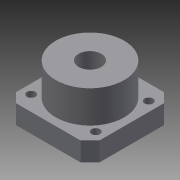
# Autodesk Inventor part: fk12
Saved by Autodesk Inventor 2014 (Build 180170000, 170)
## iProperties
Created: 2014-10-05
Part Number: fk12
Material: Generic
Document SubType Name: Modeling
Designer: Matthew
Density: 1 g/cm^3
Appearance: Default
Author: Matthew
Autodesk Inventor part; units mm, degrees
ref_plane "YZ Plane" through (0, 0, 0) normal (1, 0, 0) x (0, 1, 0)
ref_plane "XZ Plane" through (0, 0, 0) normal (0, 1, 0) x (-1, 0, 0)
ref_plane "XY Plane" through (0, 0, 0) normal (0, 0, 1) x (1, 0, 0)
sketch "Sketch1" plane through (0, 0, 0) normal (0, 0, 1) x (1, 0, 0)
  line L0 (-22, -22) -> (22, -22)
  line L1 (22, -22) -> (22, 22)
  line L2 (22, 22) -> (-22, 22)
  line L3 (-22, 22) -> (-22, -22)
  line L4 (-22, -22) -> (22, 22) construction
  line L5 (22, -22) -> (-22, 22) construction
  point P0 (0, 0)
  point P1 (0, 0)
  dimension "a" = 44
  dimension "d10" = 22
  dimension "d11" = 22
  dimension "d15" = 44
  constraints: 12 end point, 2 parallel, 1 coincident, 1 horizontal, 1 perpendicular
  measures "a" distance of L1.end L2.end
  measures "d10" distance from line of point (0, 0) L1
  measures "d11" distance from line of point (0, 0) L2
  measures "d15" distance of L2.end L0.start
extrude "Extrusion1" add sketch "Sketch1" along normal blind 10
sketch "Sketch2" plane through (0, 0, 10) normal (0, 0, 1) x (1, 0, 0)
  circle A0 centre (0, 0) radius 18
  dimension "dg6" = 36
  constraints: 1 centre point, 1 coincident
  measures "dg6" diameter of A0
extrude "Extrusion2" add sketch "Sketch2" along normal blind 17
sketch "Sketch3" plane through (0, 0, 27) normal (0, 0, 1) x (1, 0, 0)
  circle A0 centre (0, 0) radius 18 projected
  circle A1 centre (0, 0) radius 6
  dimension "d1" = 12
  constraints: 1 centre point, 1 coincident
  measures "d1" diameter of A1
extrude "Extrusion3" cut sketch "Sketch3" against normal through all contours A1
chamfer "Chamfer1" distance 5 angle 45 4 edges at (22, 22, 5) (22, -22, 5) (-22, -22, 5) (-22, 22, 5)
sketch "Sketch4" plane through (0, 0, 0) normal (0, 0, -1) x (-1, 0, 0)
  circle A0 centre (0, 0) radius 6 projected
  circle A1 centre (0, 0) radius 22 construction
  point P0 (17, 13.9642)
  point P1 (-17, -13.9642)
  point P2 (-17, 13.9642)
  point P3 (17, -13.9642)
  dimension "d16" = 44
  dimension "d17" = 34
  constraints: 4 point on circle, 2 horizontal alignment, 2 vertical alignment, 1 centre point, 1 coincident
  measures "d16" diameter of A1
  measures "d17" distance of A1.start point (-17, 13.964)
hole "Hole1" at (-17, 13.9642, 0) at (17, -13.9642, 0) at (17, 13.9642, 0) at (-17, -13.9642, 0) direction (0, 0, 1) diameter 4.5 end through all
sketch "Sketch5" plane through (0, 0, 0) normal (0, 0, -1) x (-1, 0, 0)
  circle A0 centre (-17, 13.9642) radius 2.25 projected
  circle A1 centre (17, 13.9642) radius 2.25 projected
  circle A2 centre (-17, -13.9642) radius 2.25 projected
  circle A3 centre (17, -13.9642) radius 2.25 projected
  constraints: 4 coincident
hole "Hole2" at (17, 13.9642, 0) at (-17, 13.9642, 0) at (-17, -13.9642, 0) at (17, -13.9642, 0) direction (0, 0, 1) diameter 8 depth 4
equation "\"d10\" = 0.5 * a"
equation "\"d11\" = 0.5 * a"
equation "\"d15\" = a"
body "Solid1"
